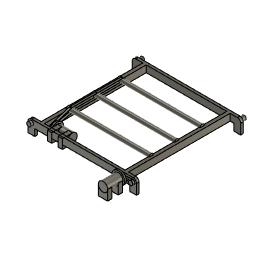
OMNI TRED FRAME v9 (Autodesk Fusion 360 design; units mm, degrees)
Autodesk Fusion 360 part; units mm, degrees
note: some values were not read from the file. Set by a fixed rule: which sketch regions a step uses.
sketch "Sketch1" plane through (0, 0, 0) normal (0, 1, 0) x (1, 0, 0)
  circle A0 centre (0, 0) radius 75
  line L0 (0, 0) -> (-1200, 0)
  circle A1 centre (-1200, 0) radius 75
  dimension "d1" = 150
  dimension "d2" = 1200
  dimension "d3" = 150
  constraint coincident A0.centre L0.start
  constraint horizontal L0
  constraint coincident L0.end A1.centre
  measures "d1" diameter of A0
  measures "d2" distance of A0.centre L0.end
  measures "d3" diameter of A1
sketch "Sketch2" plane through (0, 0, 0) normal (0, -1, 0) x (1, 0, 0)
  circle A0 centre (-1200, 0) radius 75
  circle A1 centre (-1200, 0) radius 25
  circle A2 centre (0, 0) radius 25
  dimension "d6" = 50
  constraint concentric A0 A1
  constraint coincident A2.centre origin
  measures "d6" diameter of A2
extrude "Extrude2" add sketch "Sketch2" along normal blind 60 contours A1 | A2 makes body 1 at (24.8758, -40, -2.4892) makes body 2 at (-1193.229, -40, 24.0656)
sketch "Sketch3" plane through (0, 0, 0) normal (0, -1, 0) x (1, 0, 0)
  circle A0 centre (-1200, 0) radius 25
  circle A1 centre (-1200, 0) radius 75
  circle A2 centre (-1200, 0) radius 40
  circle A3 centre (0, 0) radius 40
  line L0 (-1200, 40) -> (0, 40)
  line L1 (0, -40) -> (-1200, -40)
  line L2 (-1240, 0) -> (-1240, -120)
  line L3 (-1160, 0) -> (-1160, -120)
  line L4 (-1160, -120) -> (-1240, -120)
  line L5 (40, 0) -> (40, -120)
  line L6 (-40, 0) -> (-40, -120)
  line L7 (-40, -120) -> (40, -120)
  dimension "d9" = 80
  dimension "d10" = 80
  dimension "d11" = 120
  dimension "d12" = 120
  constraint concentric A0 A2
  constraint coincident A3.centre origin
  constraint coincident A2 L0.start
  constraint coincident A3 L0.end
  constraint tangent A3 L0
  constraint horizontal L0
  constraint coincident A3 L1.start
  constraint coincident A2 L1.end
  constraint tangent A2 L1
  constraint parallel L0 L1
  constraint coincident A2 L2.start
  constraint tangent A2 L2
  constraint vertical L2
  constraint coincident A2 L3.start
  constraint tangent A2 L3
  constraint vertical L3
  constraint perpendicular L2 L4
  constraint coincident A3 L5.start
  constraint vertical L5
  constraint coincident A3 L6.start
  constraint tangent A3 L6
  constraint vertical L6
  constraint perpendicular L5 L7
  measures "d9" diameter of A2
  measures "d10" diameter of A3
  measures "d11" distance of L5.start L5.end
  measures "d12" distance of L6.start L6.end
extrude "Extrude3" add sketch "Sketch3" along normal blind 30 separate body contours A1 A2 L0 L1 L3 | A1 A3 L0 L1 L6 | A1 A2 L1 L2 L3 | A1 L2 L3 L4 | A2 | A3 | A3 L1 L6 | A3 L1 L5 L6 L7 | A2 L1 L3 makes body 3
sketch "Sketch4" plane through (0, 0, 0) normal (0, 1, 0) x (1, 0, 0)
  circle A0 centre (0, 0) radius 55
  circle A1 centre (0, 0) radius 75
  circle A2 centre (0, 0) radius 15
  dimension "d15" = 110
  dimension "d17" = 150
  dimension "d18" = 30
  constraint coincident A0.centre A1.centre
  constraint concentric A0 A1
  constraint concentric A1 A2
  measures "d15" diameter of A0
  measures "d17" diameter of A1
  measures "d18" diameter of A2
extrude "Extrude4" add sketch "Sketch4" along normal blind 200 separate body contours A0 | A2 makes body 4
extrude "Extrude5" add sketch "Sketch4" along normal blind 20 contours A0 | A1 bodies 4
extrude "Extrude6" add sketch "Sketch4" against normal blind 25 contours A2 bodies 4
move_body "Move1" bodies 4 to x (-1, 0, 0) y (0, -1, 0) z (0, 0, 1) at (-125, -60, 0)
sketch "Sketch5" plane through (0, -260, 0) normal (0, -1, 0) x (1, 0, 0)
  circle A0 centre (-125, 0) radius 55
  line L0 (-125, 0) -> (-70, 0)
  line L1 (-70, 0) -> (-70, -120)
  line L2 (-125, 0) -> (-180, 0)
  line L3 (-180, 0) -> (-180, -120)
  line L4 (-180, -120) -> (-70, -120)
  dimension "d25" = 120
  dimension "d26" = 120
  constraint coincident A0.centre L0.start
  constraint coincident A0 L0.end
  constraint horizontal L0
  constraint perpendicular L0 L1
  constraint coincident A0 L2.end
  constraint parallel L0 L2
  constraint perpendicular L2 L3
  measures "d25" distance of L0.end L1.end
  measures "d26" distance of L2.end L3.end
extrude "Extrude7" add sketch "Sketch5" against normal blind 50 separate body contours A0 L1 L3 L4 makes body 5
copy_body "CopyPasteBodies1" bodies 5 makes body 6
move_body "Move2" bodies 6 to x (1, 0, 0) y (0, 1, 0) z (0, 0, 1) at (0, 125, 0)
sketch "Sketch6" plane through (0, -60, 0) normal (0, -1, 0) x (1, 0, 0)
  line L0 (-126.28, 15.9487) -> (-2.08, 25.9167)
  line L1 (-125, 0) -> (0, 0)
  line L2 (-2.08, -25.9167) -> (-126.28, -15.9487)
  arc A0 (-126.2, 14.9519) -> (-126.2, -14.9519) centre (-125, 0) ccw
  arc A1 (-126.28, 15.9487) -> (-125, -16.0514) centre (-124.9979, -0.0257) ccw
  arc A2 (-2, -24.9199) -> (-2, 24.9199) centre (0, 0) ccw
  arc A3 (-2.08, -25.9167) -> (-2.08, 25.9167) centre (0, 0) ccw
  line L3 (-126.2, 14.9519) -> (-2, 24.9199)
  line L4 (-2, -24.9199) -> (-126.2, -14.9519)
  dimension "d33" = 125
  constraint coincident L1.end A2.centre
  constraint horizontal L1
  constraint coincident L2 A1.end
  constraint tangent A2 L3
  constraint tangent A0 L4
  measures "d33" distance of L1.start L1.end
extrude "Extrude8" add sketch "Sketch6" against normal blind 25 separate body makes body 7
sketch "Sketch7" plane through (0, 0, 0) normal (0, 1, 0) x (-1, 0, 0)
  circle A0 centre (1200, 0) radius 25
  line L0 (40, -120) -> (40, -40)
  line L1 (40, -40) -> (1160, -40)
  line L2 (1160, -40) -> (1160, -120)
  line L3 (1160, -120) -> (1240, -120)
  line L4 (1240, -120) -> (1240, 0)
  arc A1 (1240, 0) -> (1200, 40) centre (1200, 0) ccw
  line L5 (1200, 40) -> (0, 40)
  arc A2 (0, 40) -> (-40, 0) centre (0, 0) ccw
  line L6 (-40, 0) -> (-40, -120)
  line L7 (-40, -120) -> (40, -120)
  line L8 (1075, 0) -> (125, 0)
  line L9 (1075, 0) -> (1075, 40)
  line L10 (1075, 40) -> (1115, 40)
  line L11 (1115, 40) -> (1115, -40)
  line L12 (1115, -40) -> (1075, -40)
  line L13 (1075, -40) -> (1075, 40)
  line L14 (600, 0) -> (600, 25) construction
  line L15 (125, 0) -> (125, 40) construction
  line L16 (85, 40) -> (85, -40)
  line L17 (85, -40) -> (125, -40)
  line L18 (125, -40) -> (125, 40)
  line L19 (125, 40) -> (85, 40)
  dimension "d36" = 40
  dimension "d37" = 40
  dimension "d38" = 80
  dimension "d39" = 40
  dimension "d40" = 80
  dimension "d44" = 40
  constraint parallel L1 L8
  constraint perpendicular L8 L9
  constraint horizontal L10
  constraint vertical L11
  constraint horizontal L12
  constraint vertical L13
  constraint midpoint L8 L14.start
  constraint perpendicular L8 L14
  constraint perpendicular L8 L15
  constraint vertical L16
  constraint horizontal L17
  constraint perpendicular L5 L18
  constraint perpendicular L16 L19
  measures "d36" distance of L8.start L9.end
  measures "d37" distance of L9.end L10.end
  measures "d38" distance of L9.end L12.end
  measures "d39" distance of L15.end L16.start
  measures "d40" distance of L15.end L17.end
  measures "d44" distance of L8.end L15.end
extrude "Extrude9" add sketch "Sketch7" along normal blind 1200 contours L1 L5 L16 L17 L18 L19 | L1 L5 L9 L10 L11 L12 L13 bodies 3
copy_body "CopyPasteBodies2" bodies 4 5 6 makes body 8 makes body 9 makes body 10
move_body "Move3" bodies 8 9 10 to x (0, 1, 0) y (-1, 0, 0) z (0, 0, 1) at (-1110, 200, 0)
sketch "Sketch8" plane through (-1075, 0, 0) normal (1, 0, 0) x (0, 1, 0)
  line L0 (0, 40) -> (0, -40)
  line L1 (0, -40) -> (1200, -40)
  line L2 (1200, -40) -> (1200, 40)
  line L3 (1200, 40) -> (0, 40)
  line L4 (0, 0) -> (1200, 0)
  circle A0 centre (600, 0) radius 25
  line L5 (600, 0) -> (250, 0)
  line L6 (600, 0) -> (950, 0)
  circle A1 centre (950, 0) radius 25
  circle A2 centre (250, 0) radius 25
  line L7 (0, 0) -> (250, 0)
  line L8 (950, 0) -> (1200, 0)
  line L9 (0, 0) -> (250, 0)
  line L10 (0, 0) -> (600, 0)
  dimension "d43" = 50
  dimension "d45" = 350
  dimension "d46" = 350
  dimension "d47" = 50
  dimension "d48" = 50
  dimension "d71" = 250
  dimension "d72" = 250
  constraint coincident L4.start L7.start
  constraint midpoint L2 L4.end
  constraint coincident L4 A0.centre
  constraint coincident A0.centre L5.start
  constraint perpendicular L0 L5
  constraint parallel L4 L6
  constraint coincident L6.end A1.centre
  constraint coincident L5.end A2.centre
  constraint perpendicular L2 L8
  measures "d43" diameter of A0
  measures "d45" distance of A0.centre L5.end
  measures "d46" distance of A0.centre L6.end
  measures "d47" diameter of A1
  measures "d48" diameter of A2
  measures "d71" distance of L4.start L5.end
  measures "d72" distance of L4.end L6.end
sketch "Sketch10" plane through (0, 1200, 0) normal (0, 1, 0) x (-1, 0, 0)
  line L0 (125, 40) -> (85, 40)
  line L1 (85, 40) -> (85, -40)
  line L2 (85, -40) -> (125, -40)
  line L3 (125, -40) -> (125, 40)
  line L4 (0, 0) -> (1200, 0)
  circle A0 centre (0, 0) radius 40
  circle A1 centre (1200, 0) radius 40
  line L5 (40, 0) -> (40, -120)
  line L6 (-40, 0) -> (-40, -120)
  line L7 (-40, -120) -> (40, -120)
  line L8 (1160, 0) -> (1160, -120)
  line L9 (1240, 0) -> (1240, -120)
  line L10 (1240, -120) -> (1160, -120)
  line L11 (0, -40) -> (1200, -40)
  line L12 (1200, 40) -> (0, 40)
  dimension "d62" = 80
  dimension "d63" = 80
  constraint coincident L4.start A0.centre
  constraint horizontal L4
  constraint coincident L4.end A1.centre
  constraint coincident L4 L5.start
  constraint coincident A0 L5.start
  constraint tangent A0 L5
  constraint coincident A0 L6.start
  constraint tangent A0 L6
  constraint vertical L6
  constraint perpendicular L5 L7
  constraint coincident A1 L8.start
  constraint coincident L4 L8.start
  constraint tangent A1 L8
  constraint coincident A1 L9.start
  constraint tangent A1 L9
  constraint vertical L9
  constraint perpendicular L9 L10
  constraint coincident A0 L11.start
  constraint coincident A1 L11.end
  constraint tangent A1 L11
  constraint perpendicular L8 L11
  constraint coincident A1 L12.start
  constraint coincident A0 L12.end
  constraint tangent A0 L12
  constraint parallel L11 L12
  measures "d62" diameter of A0
  measures "d63" diameter of A1
extrude "Extrude12" add sketch "Sketch10" along normal blind 30 bodies 3
sketch "Sketch11" plane through (0, 1230, 0) normal (0, 1, 0) x (-1, 0, 0)
  arc A0 (1240, 0) -> (1200, 40) centre (1200, 0) ccw
  line L0 (1200, 40) -> (0, 40)
  arc A1 (0, 40) -> (-40, 0) centre (0, 0) ccw
  line L1 (-40, 0) -> (-40, -120)
  line L2 (-40, -120) -> (40, -120)
  line L3 (40, -120) -> (40, -40)
  line L4 (40, -40) -> (1160, -40)
  line L5 (1160, -40) -> (1160, -120)
  line L6 (1160, -120) -> (1240, -120)
  line L7 (1240, -120) -> (1240, 0)
  circle A2 centre (0, 0) radius 25
  line L8 (0, 0) -> (1200, 0)
  circle A3 centre (1200, 0) radius 25
  dimension "d66" = 50
  dimension "d67" = 1200
  dimension "d68" = 50
  constraint coincident A1.centre A2.centre
  constraint horizontal L8
  constraint coincident A0.centre L8.end
  measures "d66" diameter of A2
  measures "d67" distance of A1.centre A0.centre
  measures "d68" diameter of A3
extrude "Extrude13" add sketch "Sketch11" along normal blind 50 contours A2 | A3 bodies 3
move_body "Move4" bodies 8 9 10 to x (1, 0, 0) y (0, 0, -1) z (0, 1, 0) at (30, 75, 55)
sketch "Sketch12" plane through (-1075, 0, 0) normal (1, 0, 0) x (0, 1, 0)
  line L0 (0, 40) -> (0, -40)
  line L1 (0, -40) -> (1200, -40)
  line L2 (1200, -40) -> (1200, 40)
  line L3 (1200, 40) -> (0, 40)
  line L4 (0, 0) -> (1200, 0)
  line L5 (600, 0) -> (600, 40)
  line L6 (600, 0) -> (300, 0)
  line L7 (600, 0) -> (900, 0)
  line L8 (300, 0) -> (300, 40)
  line L9 (900, 0) -> (900, 40)
  circle A0 centre (300, 40) radius 25
  circle A1 centre (600, 40) radius 25
  circle A2 centre (900, 40) radius 25
  dimension "d77" = 300
  dimension "d78" = 300
  dimension "d79" = 50
  dimension "d80" = 50
  dimension "d81" = 50
  constraint coincident L4.start origin
  constraint midpoint L2 L4.end
  constraint midpoint L4 L5.start
  constraint midpoint L3 L5.end
  constraint coincident L4 L6.end
  constraint perpendicular L5 L6
  constraint coincident L4 L7.end
  constraint perpendicular L5 L7
  constraint coincident L3 L8.end
  constraint perpendicular L3 L8
  constraint coincident L3 L9.end
  constraint perpendicular L3 L9
  constraint coincident L8.end A0.centre
  constraint coincident L5.end A1.centre
  constraint coincident L9.end A2.centre
  measures "d77" distance of L5.start L6.end
  measures "d78" distance of L5.start L7.end
  measures "d79" diameter of A0
  measures "d80" diameter of A1
  measures "d81" diameter of A2
extrude "Extrude14" add sketch "Sketch12" along normal blind 30 and the other way blind 20 separate body contours L3 A0 | L3 L8 A0 | L3 L8 A0 | L3 A1 | L3 L5 A1 | L3 L5 A1 | L3 L9 A2 | L3 L9 A2 | L3 A2 makes body 11 at (-1078.3333, 324.8758, 37.5108) makes body 12 at (-1078.3333, 603.1086, 64.806) makes body 13 at (-1078.3333, 903.1086, 64.806)
sketch "Sketch13" plane through (-1075, 0, 0) normal (1, 0, 0) x (0, 1, 0)
  line L0 (0, 40) -> (0, -40)
  line L1 (0, -40) -> (1200, -40)
  line L2 (1200, -40) -> (1200, 40)
  line L3 (1200, 40) -> (0, 40)
  line L4 (0, 0) -> (1200, 0)
  line L5 (0, 0) -> (75, 0)
  line L6 (75, 0) -> (75, -20)
  line L7 (300, 0) -> (300, 40)
  line L8 (600, 0) -> (600, 40)
  line L9 (900, 0) -> (900, 40)
  line L10 (300, 65) -> (600, 65)
  line L11 (600, 65) -> (900, 65)
  line L12 (78.277, -34.6377) -> (300, 15)
  line L13 (300, 15) -> (600, 15)
  line L14 (600, 15) -> (900, 15)
  line L15 (290.0112, 62.9178) -> (70.5252, -5.683)
  line L16 (67.8569, -5.683) -> (292.2068, 64.8045)
  line L17 (300, 66) -> (600, 66)
  line L18 (600, 66) -> (900, 66)
  line L19 (900, 14) -> (600, 14)
  line L20 (600, 14) -> (300, 14)
  line L21 (300, 14) -> (78.4971, -35.6131)
  arc A0 (70.5252, -5.683) -> (78.277, -34.6377) centre (75, -20) ccw
  arc A1 (67.8569, -5.683) -> (78.4971, -35.6131) centre (75, -20) ccw
  arc A2 (900, 15) -> (900, 65) centre (900, 40) ccw
  arc A3 (900, 14) -> (900, 66) centre (900, 40) ccw
  line L22 (290.0112, 62.9178) -> (300, 65)
  line L23 (300, 66) -> (290.0112, 64.1147)
  dimension "d86" = 90
  dimension "d87" = 20
  constraint coincident L4.start L5.start
  constraint midpoint L2 L4.end
  constraint coincident L4 L5.end
  constraint perpendicular L4 L6
  constraint coincident L4 L7.start
  constraint coincident L3 L7.end
  constraint perpendicular L4 L7
  constraint midpoint L4 L8.start
  constraint midpoint L3 L8.end
  constraint coincident L4 L9.start
  constraint coincident L3 L9.end
  constraint perpendicular L3 L9
  constraint parallel L3 L10
  constraint parallel L10 L11
  constraint coincident L7 L12.end
  constraint coincident L8 L13.end
  constraint coincident L9 L14.end
  constraint parallel L11 L17
  constraint parallel L11 L18
  constraint coincident L9 L19.start
  constraint coincident L8 L19.end
  constraint parallel L19 L20
  constraint tangent L15 A0
  constraint tangent L14 A2
  constraint coincident L16 L23.end
  measures "d86" angle of L5 L6
  measures "d87" distance of L5.end L6.end
extrude "Extrude15" add sketch "Sketch13" along normal blind 25 contours L3 L10 L11 L15 L16 L17 L18 A2 A3 L22 L23 | L3 L4 L15 L16 | L4 L6 L15 L16 | L4 L6 L12 L15 L16 L21 A0 A1 | L7 L8 L13 L20 | L4 L7 L12 L21 | L8 L9 L14 L19 | L3 L9 A2 A3 bodies 11 8 9 10 3 13 12
extrude "Extrude19" add 3 faces at (-1045, 601.799, 32.2427) (-1045, 305.1957, 35.1791) (-1045, 901.799, 32.2427) along direction (1, 0, 0) blind 930 on bodies 11 bodies 11
